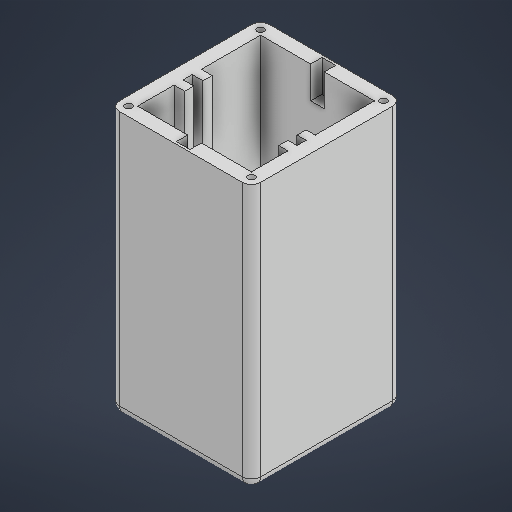
# Autodesk Inventor part: CajaNodoReceptor
Saved by Autodesk Inventor 2027.1 (Build 311270010, 270A)
## iProperties
Created: 2026-09-09
Part Number: CajaNodoReceptor
Material: Genérico
Document SubType Name: Sheet Metal
Designer: marco
Density: 1 g/cm^3
Sheet Metal Rule: Por defecto_mm
Appearance: Valor por defecto
Author: marco
Autodesk Inventor part; units mm, degrees
ref_plane "YZ Plane" through (0, 0, 0) normal (1, 0, 0) x (0, 1, 0)
ref_plane "XZ Plane" through (0, 0, 0) normal (0, 1, 0) x (-1, 0, 0)
ref_plane "XY Plane" through (0, 0, 0) normal (0, 0, 1) x (1, 0, 0)
sketch "Boceto1" plane through (0, 0, 0) normal (0, 1, 0) x (-1, 0, 0)
  line L0 (0, 0) -> (-31, 0)
  line L1 (-31, 0) -> (-31, -33)
  line L2 (-31, -33) -> (0, -33)
  line L3 (0, -33) -> (0, 0)
  line L4 (0, -33) -> (0, -30)
  line L5 (0, -30) -> (0, -15)
  line L6 (0, -15) -> (0, -13)
  line L7 (0, -13) -> (0, -3)
  line L8 (0, -3) -> (0, 0)
  line L9 (0, -30) -> (-31, -30)
  line L10 (0, -15) -> (-31, -15)
  line L11 (0, -13) -> (-31, -13)
  line L12 (0, -3) -> (-31, -3)
  line L13 (0, -33) -> (-3, -33)
  line L14 (0, -33) -> (-3, -33)
  line L15 (-3, -33) -> (-3, 0)
  line L16 (-31, -33) -> (-28, -33)
  line L17 (-28, -33) -> (-28, 0)
  line L18 (-3, -15) -> (-3, -17)
  line L19 (-3, -17) -> (-5.3627, -17)
  line L20 (-5.3627, -17) -> (-5.3627, -15)
  line L21 (-5.3627, -13) -> (-5.3627, -11)
  line L22 (-5.3627, -11) -> (-3, -11)
  line L23 (-28, -15) -> (-26, -15)
  line L24 (-26, -15) -> (-26, -17)
  line L25 (-26, -17) -> (-28, -17)
  line L26 (-26, -13) -> (-26, -11)
  line L27 (-26, -11) -> (-28, -11)
  point P0 (-3, -30)
  point P1 (-28, -30)
  point P2 (-28, -13)
  point P3 (-28, -3)
  point P4 (-3, -3)
  point P5 (-3, -13)
  dimension "d0" = 31
  dimension "d1" = 33
  dimension "d2" = 3
  dimension "d3" = 15
  dimension "d4" = 2
  dimension "d5" = 10
  dimension "d6" = 3
  dimension "d7" = 3
  dimension "d8" = 2
  dimension "d9" = 2
  dimension "d10" = 2
  dimension "d11" = 2
  dimension "d12" = 2
  constraints: 56 end point, 28 point on line, 13 perpendicular, 2 collinear, 2 parallel, 1 horizontal
  measures "d0" distance of L2.end L1.end
  measures "d1" distance of L1.end L0.end
  measures "d2" distance of L2.end L4.end
  measures "d3" distance of L4.end L5.end
  measures "d4" distance of L5.end L6.end
  measures "d5" distance of L6.end L7.end
  measures "d6" distance of L2.end L13.end
  measures "d7" distance of L1.end L16.end
  measures "d8" distance of L18.start L18.end
  measures "d9" distance of L21.start L21.end
  measures "d10" distance of L23.start L23.end
  measures "d11" distance of L23.end L24.end
  measures "d12" distance of L26.start L26.end
extrude "Extrusión1" add sketch "Boceto1" along normal blind 58 contours L3 L12 L15 L0 | L15 L12 L17 L0 | L3 L11 L15 L12 | L17 L12 L1 L0 | L3 L10 L15 L11 | L17 L11 L1 L12 | L15 L11 L21 L22 | L3 L9 L15 L10 | L27 L26 L11 L17 | L3 L2 L15 L9 | L15 L19 L20 L10 | L11 L17 L10 L1 | L15 L2 L17 L9 | L10 L17 L9 L1 | L10 L24 L25 L17 | L17 L2 L1 L9
sketch "Boceto2" plane through (31, 0, 0) normal (1, 0, 0) x (0, 0, -1)
  line L0 (33, 0) -> (33, 58) projected
  line L1 (0, 0) -> (0, 58) projected
  line L2 (33, 0) -> (0, 0)
  line L3 (0, 0) -> (0, 3)
  line L4 (0, 3) -> (33, 3)
  line L5 (33, 3) -> (33, 0)
  dimension "d15" = 3
  constraints: 8 end point, 2 parallel, 1 horizontal, 1 perpendicular, 1 point on line
  measures "d15" distance of L2.end L3.end
extrude "Extrusión2" add sketch "Boceto2" against normal up to surface (28 mm away)
fillet "Empalme1" radius 2 10 edges at (31, 29, 0) (15.5, 0, 0) (31, 0, -16.5) (31, 29, -33) (15.5, 0, -33) (0, 0, -16.5) (0, 29, 0) (0, 29, -33) (15.5, 3, -3) (15.5, 3, -30)
sketch "Boceto4" plane through (0, 58, 0) normal (0, 1, 0) x (1, 0, 0)
  line L0 (0, 31) -> (2, 31) projected
  circle A0 centre (2, 31) radius 0.75
  line L1 (29, 31) -> (31, 31) projected
  circle A1 centre (29, 31) radius 0.75
  line L2 (2, 0) -> (2, 2) projected
  circle A2 centre (2, 2) radius 0.75
  line L3 (2, 2) -> (29, 2) projected
  circle A3 centre (29, 2) radius 0.75
  line L4 (2, 31) -> (15.5, 31)
  line L5 (29, 31) -> (2, 31) projected
  line L6 (14, 29.5) -> (17, 29.5)
  line L7 (17, 29.5) -> (17, 32.5)
  line L8 (17, 32.5) -> (14, 32.5)
  line L9 (14, 32.5) -> (14, 29.5)
  line L10 (14, 29.5) -> (17, 32.5) construction
  line L11 (17, 29.5) -> (14, 32.5) construction
  line L12 (14, 0.5) -> (17, 0.5)
  line L13 (17, 0.5) -> (17, 3.5)
  line L14 (17, 3.5) -> (14, 3.5)
  line L15 (14, 3.5) -> (14, 0.5)
  line L16 (14, 0.5) -> (17, 3.5) construction
  line L17 (17, 0.5) -> (14, 3.5) construction
  point P0 (0, 0)
  point P1 (15.5, 2)
  dimension "d19" = 1.5
  dimension "d20" = 1.5
  dimension "d21" = 1.5
  dimension "d22" = 1.5
  dimension "d23" = 3
  dimension "d24" = 3
  dimension "d25" = 3
  dimension "d26" = 3
  constraints: 26 end point, 6 midpoint, 4 centre point, 4 parallel, 2 horizontal, 2 perpendicular
  measures "d19" diameter of A0
  measures "d20" diameter of A1
  measures "d21" diameter of A2
  measures "d22" diameter of A3
  measures "d23" distance of L8.end L7.end
  measures "d24" distance of L7.end L6.end
  measures "d25" distance of L14.end L13.end
  measures "d26" distance of L13.end L12.end
extrude "Extrusión3" cut sketch "Boceto4" against normal blind 7
equation "\"Radio_pliegue\" = Grosor"
equation "\"Anchura_desahogo_plegado\" = Grosor"
equation "\"Profundidad_desahogo_plegado\" = 0.5 * Grosor"
equation "\"Tamaño_destalonado\" = 4 * Grosor"
equation "\"Remanente_mínimo\" = 2 * Grosor"
equation "\"Radiodetransición\" = Radio_pliegue"
equation "\"Tamaño_de_radio_de_Jacobi\" = Radio_pliegue"
equation "\"TamañoSeparación\" = Grosor"
equation "\"Grosor\" = 0.5"
